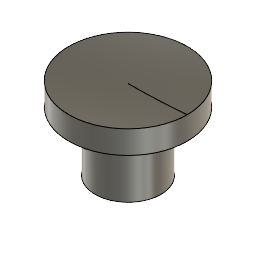
glowka_pada (Autodesk Fusion 360 design; units mm, degrees)
part number: 2026-01-04-21-26-33-544
Autodesk Fusion 360 part; units mm, degrees
sketch "Szkic1" plane through (0, 0, 0) normal (0, 1, 0) x (1, 0, 0)
  line L0 (0, 0) -> (5, 0)
  line L1 (5, 0) -> (5, -9)
  line L2 (5, -9) -> (9, -9)
  line L3 (9, -9) -> (9, -12.5)
  line L4 (0, -29.9609) -> (0, -12.1) construction
  line L5 (0, 0) -> (0, 2.9959) construction
  spline S0 degree 5 poles (9, -12.5) (8.8201, -12.4844) (8.4604, -12.4539) (7.9207, -12.4102) (7.2011, -12.3559) (6.3015, -12.2952) (5.4017, -12.2423) (4.5018, -12.1979) (3.6017, -12.1623) (2.7015, -12.1352) (1.8011, -12.1159) (1.0807, -12.1062) (0.5404, -12.1019) (0.1801, -12.1004) (0, -12.1) knots 0 0 0 0 0 0 0.1 0.2 0.3 0.4 0.5 0.6 0.7 0.8 0.9 1 1 1 1 1 1
  line L6 (0, -12.1) -> (0, 0)
  point P0 (4.5, -12.2)
  dimension "d4" = 9
  dimension "d5" = 9
  dimension "d6" = 3.5
  dimension "d10" = 4.5
  dimension "d12" = 0.4
  dimension "d13" = 0.3
  dimension "d14" = 5
  constraint coincident L0.start L5.start
  constraint horizontal L0
  constraint perpendicular L0 L1
  constraint perpendicular L1 L2
  constraint perpendicular L2 L3
  constraint coincident L0 L5.start
  constraint collinear L4 L5
  constraint vertical L4
  constraint coincident L0.start L4
  measures "d4" distance of L3 L4.end
  measures "d5" distance of L0 L2
  measures "d6" distance of L2.end L3.end
  measures "d10" horizontal distance of P0 L4.end
  measures "d12" vertical distance of L3.end L4.end
  measures "d13" vertical distance of L3.end P0
  measures "d14" distance of L0.start L1
revolve "Obrót1" add sketch "Szkic1" angle 360 about axis through (0, 0, 29.9609) along (0, 0, -1)
